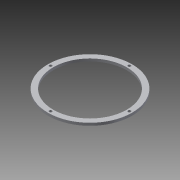
# Autodesk Inventor part: Flywheel Spacer
Saved by Autodesk Inventor 2013 (Build 170138000, 138)
## iProperties
Created: 2013-01-17
Part Number: Flywheel Spacer
Material: Aluminum 6061
Document SubType Name: Modeling
Designer: actoennies
Mass: 371.723 g
Surface Area: 230.542 cm^2
Volume: 47.3532 cm^3
Density: 7.85 g/cm^3
Author: actoennies
Autodesk Inventor part; units mm, degrees
ref_plane "YZ Plane" through (0, 0, 0) normal (1, 0, 0) x (0, 1, 0)
ref_plane "XZ Plane" through (0, 0, 0) normal (0, 1, 0) x (-1, 0, 0)
ref_plane "XY Plane" through (0, 0, 0) normal (0, 0, 1) x (1, 0, 0)
sketch "Sketch1" plane through (0, 0, 0) normal (0, 1, 0) x (-1, 0, 0)
  circle A0 centre (0, 0) radius 88.9
  circle A1 centre (0, 0) radius 101.6
  circle A2 centre (0, 0) radius 95.25 construction
  circle A3 centre (0, 95.25) radius 3.3782
  circle A4 centre (-95.25, 0) radius 3.3782
  circle A5 centre (0, -95.25) radius 3.3782
  circle A6 centre (95.25, 0) radius 3.3782
  dimension "d2" = 190.5
  dimension "d0" = 177.8
  dimension "d1" = 203.2
  dimension "d3" = 6.7564
  dimension "d6" = 360
  constraints: 6 centre point, 3 coincident, 1 vertical alignment, 11 other
  measures "d0" diameter of A0
  measures "d1" diameter of A1
  measures "d3" diameter of A3
extrude "Extrusion1" add sketch "Sketch1" along normal blind 6.35
body "Solid1"
